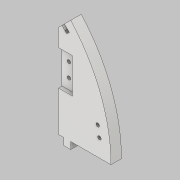
# Autodesk Inventor part: CP001
Saved by Autodesk Inventor 2017 (Build 210142000, 142)
## iProperties
Created: 2017-05-15
Part Number: CP001
Material: ABS Plastic
Document SubType Name: Modeling
Designer: zallen
Density: 1.06 g/cm^3
Appearance: Smooth - White
Mass: 127.889 g
Surface Area: 242.607 cm^2
Volume: 120.65 cm^3
Author: zallen
Autodesk Inventor part; units mm, degrees
ref_plane "YZ Plane" through (0, 0, 0) normal (1, 0, 0) x (0, 1, 0)
ref_plane "XZ Plane" through (0, 0, 0) normal (0, 1, 0) x (-1, 0, 0)
ref_plane "XY Plane" through (0, 0, 0) normal (0, 0, 1) x (1, 0, 0)
sketch "Sketch1" plane through (0, 0, 0) normal (0, 0, 1) x (1, 0, 0)
  circle A0 centre (-149.9998, -0.3235) radius 225 construction
  line L0 (0, 0) -> (0, 132.4058)
  line L1 (0, 132.4058) -> (17.5, 149.9058)
  line L2 (0, 132.4058) -> (24.7487, 132.4058) construction
  arc A1 (75, 0) -> (17.5, 149.9058) centre (-149.9998, -0.3235) ccw
  line L3 (75, 0) -> (25, 0)
  line L4 (25, 0) -> (17.5, 0)
  line L5 (0, 0) -> (7.5, 0)
  line L6 (7.5, 0) -> (7.5, -10)
  line L7 (7.5, -10) -> (17.5, -10)
  line L8 (17.5, -10) -> (17.5, 0)
  circle A2 centre (-149.9998, -0.3235) radius 200 construction
  line L9 (17.5, 149.9058) -> (17.5, 0)
  dimension "d0" = 75
  dimension "d1" = 450
  dimension "d3" = 45
  dimension "d37" = 50
  dimension "d38" = 7.5
  dimension "d39" = 7.5
  dimension "d40" = 10
  dimension "d41" = 25
  dimension "d79" = 149.9058
  constraints: 20 end point, 4 perpendicular, 4 point on circle, 3 centre point, 3 horizontal, 1 concentric, 1 equal length, 1 point on line, 1 vertical
  measures "d0" distance of L0.start L3.start
  measures "d1" diameter of A0
  measures "d3" angle of L2 L1
  measures "d37" distance of L3.start L3.end
  measures "d38" distance of L3.end L4.end
  measures "d39" distance of L0.start L5.end
  measures "d40" distance of L5.end L6.end
  measures "d41" radial gap between concentric circles of A0 A2
  measures "d79" distance of L1.end L4.end
extrude "Extrusion1" add sketch "Sketch1" along normal blind 15
sketch "Sketch2" plane through (0, 0, 15) normal (0, 0, 1) x (1, 0, 0)
  circle A0 centre (58.4678, 25) radius 2.5
  circle A1 centre (56.1283, 39.8164) radius 2.5
  line L0 (0, 132.4058) -> (0, 0) projected
  line L1 (0, 0) -> (7.5, 0) projected
  line L2 (7.5, 0) -> (7.5, -10) projected
  line L3 (7.5, -10) -> (17.5, -10) projected
  line L4 (17.5, -10) -> (17.5, 0) projected
  line L5 (17.5, 0) -> (75, 0) projected
  arc A2 (75, 0) -> (17.5, 149.9058) centre (-149.9998, -0.3235) ccw projected
  line L6 (17.5, 149.9058) -> (0, 132.4058) projected
  arc A3 (59.4404, 15) -> (16.4825, 127.6751) centre (-149.9998, -0.3235) ccw construction
  line L7 (59.4404, 15) -> (17.5, 15) construction
  line L8 (17.5, 15) -> (15, 15) construction
  line L9 (15, 15) -> (15, 126.1926) construction
  line L10 (15, 126.1926) -> (16.4825, 127.6751) construction
  circle A4 centre (11.7593, 133.5945) radius 2.5
  circle A5 centre (-149.9998, -0.3235) radius 225 construction
  circle A6 centre (-149.9998, -0.3235) radius 210 construction
  dimension "d6" = 5
  dimension "d7" = 5
  dimension "d8" = 15
  dimension "d10" = 25
  dimension "d42" = 15
  dimension "d43" = 5
  dimension "d45" = 450
  dimension "d46" = 15
  dimension "d49" = 7.4745
  constraints: 8 end point, 5 centre point, 4 point on circle, 1 concentric, 7 other
  measures "d6" diameter of A0
  measures "d7" diameter of A1
  measures "d8" distance of A0.centre A1.centre
  measures "d10" vertical distance of point (0, 0) A0.centre
  measures "d42" radial gap between concentric circles of A2 A3
  measures "d43" diameter of A4
  measures "d45" diameter of A5
  measures "d49" distance from line of L6 A4.centre
extrude "Extrusion2" cut sketch "Sketch2" against normal through all contours A0 | A1 | A4
sketch "Sketch5" plane through (0, 0, 15) normal (0, 0, 1) x (1, 0, 0)
  line L0 (5, 137.4058) -> (12.0711, 130.3347)
  line L1 (5, 137.4058) -> (15, 137.4058) construction
  line L2 (12.0711, 130.3347) -> (15.6066, 133.8703)
  line L3 (15.6066, 133.8703) -> (8.5355, 140.9413)
  line L4 (8.5355, 140.9413) -> (5, 137.4058)
  line L5 (17.5, 149.9058) -> (0, 132.4058) projected
  point P0 (0, 0)
  dimension "d29" = 10
  dimension "d30" = 45
  dimension "d31" = 5
  dimension "d32" = 10
  dimension "d33" = 90
  dimension "d34" = 5
  constraints: 10 end point, 2 perpendicular, 1 equal length, 1 horizontal, 1 point on line
  measures "d29" distance of L0.start L0.end
  measures "d30" angle of L0 L1
  measures "d31" distance of L0.end L2.end
  measures "d32" distance of L2.end L3.end
  measures "d33" angle of L3 L2
  measures "d34" horizontal distance of L0.start L5.end
extrude "Extrusion3" cut sketch "Sketch5" against normal through all
thread "Thread1" size "M5x0.8" class "6H" standard "ANSI Metric M Profile" full length
thread "Thread2" size "M5x0.8" class "6H" standard "ANSI Metric M Profile" full length
thread "Thread3" size "M5x0.8" class "6H" standard "ANSI Metric M Profile" full length
sketch "Sketch6" plane through (0, 0, 15) normal (0, 0, 1) x (1, 0, 0)
  line L0 (0, 107.4058) -> (20, 107.4058) construction
  line L1 (20, 107.4058) -> (20, 57.4058) construction
  line L2 (20, 57.4058) -> (0, 57.4058) construction
  line L3 (0, 57.4058) -> (0, 107.4058) construction
  line L4 (8.5355, 140.9413) -> (15.6066, 133.8703) construction
  line L5 (15.6066, 133.8703) -> (12.0711, 130.3347) construction
  line L6 (9.3094, 133.0964) -> (5, 137.4058) construction
  line L7 (5, 137.4058) -> (0, 132.4058) construction
  line L8 (0, 132.4058) -> (0, 0) construction
  line L9 (0, 0) -> (7.5, 0) construction
  line L10 (7.5, 0) -> (7.5, -10) construction
  line L11 (7.5, -10) -> (17.5, -10) construction
  line L12 (17.5, -10) -> (17.5, 0) construction
  line L13 (17.5, 0) -> (75, 0) construction
  arc A0 (75, 0) -> (17.5, 149.9058) centre (-149.9998, -0.3235) ccw construction
  line L14 (17.5, 149.9058) -> (8.5355, 140.9413) construction
  arc A1 (9.3094, 133.0964) -> (11.2612, 131.1446) centre (11.7593, 133.5945) ccw construction
  circle A2 centre (58.4678, 25) radius 2.5 construction
  circle A3 centre (56.1283, 39.8164) radius 2.5 construction
  circle A4 centre (10, 92.4058) radius 2.5
  circle A5 centre (10, 72.4058) radius 2.5
  line L15 (0, 132.4058) -> (0, 0) projected
  line L16 (12.0711, 130.3347) -> (11.2612, 131.1446) projected
  dimension "d50" = 20
  dimension "d51" = 50
  dimension "d52" = 25
  dimension "d53" = 5
  dimension "d54" = 5
  dimension "d55" = 20
  dimension "d56" = 15
  dimension "d57" = 10
  constraints: 8 end point, 2 centre point, 2 parallel, 1 horizontal, 1 perpendicular, 1 point on line, 1 vertical alignment
  measures "d50" distance of L1.end L2.end
  measures "d51" distance of L0.end L1.end
  measures "d52" distance of L0.start L7.end
  measures "d53" diameter of A4
  measures "d54" diameter of A5
  measures "d55" distance of A5.centre A4.centre
  measures "d56" distance from line of L0 A4.centre
  measures "d57" distance from line of L3 A4.centre
extrude "Extrusion4" cut sketch "Sketch6" against normal through all
thread "Thread4" size "M5x0.8" class "6H" standard "ANSI Metric M Profile" full length
thread "Thread5" size "M5x0.8" class "6H" standard "ANSI Metric M Profile" full length
sketch "Sketch9" plane through (0, 0, 15) normal (0, 0, 1) x (1, 0, 0)
  line L0 (0, 132.4058) -> (0, 0) projected
  line L1 (0, 107.4058) -> (20, 107.4058)
  line L2 (20, 107.4058) -> (20, 57.4058)
  line L3 (20, 57.4058) -> (0, 57.4058)
  line L4 (0, 57.4058) -> (0, 107.4058)
  dimension "d74" = 20
  dimension "d75" = 50
  dimension "d76" = 25
  constraints: 8 end point, 2 parallel, 1 horizontal, 1 perpendicular, 1 point on line
  measures "d74" distance of L2.end L3.end
  measures "d75" distance of L1.end L2.end
  measures "d76" distance of L1.start L0.start
extrude "Extrusion7" cut sketch "Sketch9" against normal blind 5
body "Solid1"
